# Autodesk Inventor part: Synchronous Pulley2
Saved by Autodesk Inventor 2013 (Build 170138000, 138)
## iProperties
Created: 2013-09-18
Part Number: Synchronous Pulley2
Material: Steel
Document SubType Name: Modeling
Designer: Ian
Density: 7.85 g/cm^3
Mass: 1317.92 g
Surface Area: 246.578 cm^2
Volume: 167.887 cm^3
CustomPartVersion: 1
Author: Ian
Autodesk Inventor part; units mm, degrees
ref_plane "YZ Plane" through (0, 0, 0) normal (1, 0, 0) x (0, 1, 0)
ref_plane "XZ Plane" through (0, 0, 0) normal (0, 1, 0) x (-1, 0, 0)
ref_plane "XY Plane" through (0, 0, 0) normal (0, 0, 1) x (1, 0, 0)
sketch "Pulley Sketch" plane through (0, 0, 0) normal (0, 0, 1) x (1, 0, 0)
  circle A0 centre (0, 0) radius 44.4679 construction
  circle A1 centre (0, 0) radius 43.7821
  circle A2 centre (0, 0) radius 40.7341
  line L0 (-3.1632, 43.6677) -> (-2.0955, 40.7341)
  line L1 (-2.0955, 40.7341) -> (2.0955, 40.7341)
  line L2 (2.0955, 40.7341) -> (3.1632, 43.6677)
  line L3 (0, 0) -> (0, 43.7821) construction
  point P0 (0, 40.7341)
  dimension "d0" = 88.9358
  dimension "d1" = 0.6858
  dimension "d2" = 3.048
  dimension "d3" = 40
  dimension "d4" = 4.191
  constraints: 8 end point, 3 coincident, 3 point on circle, 2 centre point, 1 horizontal, 1 midpoint, 1 point on line, 1 vertical, 1 vertical alignment, 3 other
  measures "d0" diameter of A0
  measures "d1" radial gap between concentric circles of A0 A1
  measures "d3" angle of L2 L0
  measures "d4" distance of L0.end L1.end
extrude "Base Body" add sketch "Pulley Sketch" along normal mid plane 26.67 contours A2 | A1 L0 L1 L2 | L2 L1 L0 A1
extrude "Tooth" cut sketch "Pulley Sketch" along normal through all both and the other way through all contours L2 L1 L0 A1 picked at (0, 42.7576)
fillet "Tooth Fillet" radius 1.6002 2 edges at (2.0955, 40.7341, 0) (-2.0955, 40.7341, 0)
fillet "Tooth Fillet" radius 1.6002 4 edges at (-3.1632, 43.6677, 6.6675) (-3.1632, 43.6677, -6.6675) (3.1632, 43.6677, 6.6675) (3.1632, 43.6677, -6.6675)
pattern_circular "Teeth" count 22 over 360 about axis through (0, 0, -10) along (0, 0, 1) of "Tooth", "Tooth Fillet"
pulley flange "Left flange" diameter 87.5642 height 2.032 thickness 1.27 bend angle 10 centre (0, 0, -13.335) toward (0, 0, -1)
pulley flange "Right flange" diameter 87.5642 height 2.032 thickness 1.27 bend angle 10 centre (0, 0, 13.335) toward (0, 0, 1)
equation "\"d1\" = da_a"
equation "\"d2\" = da_hg"
equation "\"d3\" = 2 * da_fi"
equation "\"d4\" = da_bw"
equation "\"d5\" = da_bf"
equation "\"d7\" = da_bf"
equation "\"d9\" = da_rb"
equation "\"d10\" = da_rt"
equation "\"da_pb\" = 12.7"
equation "\"da_fi\" = 20deg"
equation "\"da_hg\" = 3.048"
equation "\"da_bw\" = 4.191"
equation "\"da_rb\" = 1.6002"
equation "\"da_rt\" = 1.6002"
equation "\"da_a\" = 0.6858"
equation "\"da_bf\" = 26.67"
equation "\"da_wf\" = 1.27"
equation "\"da_hf\" = 2.032"
body "Solid1"
